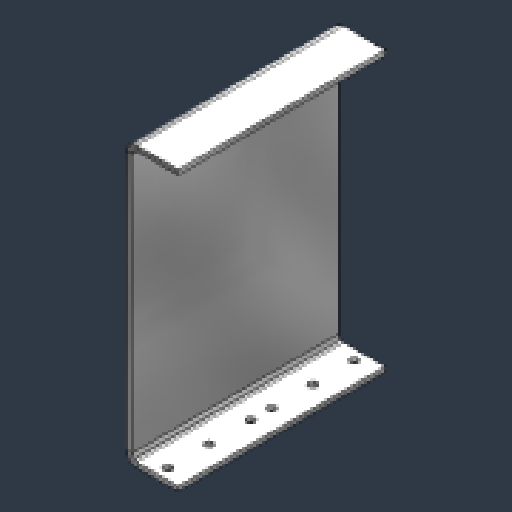
# Autodesk Inventor part: trough_back_support
Saved by Autodesk Inventor 2024.3 (Build 283343000, 343)
## iProperties
Created: 2025-03-03
Part Number: trough_back_support
Material: Aluminum 6061
Document SubType Name: Sheet Metal
Designer: marcu
Mass: 478.765 g
Surface Area: 1202.18 cm^2
Volume: 177.321 cm^3
Density: 2.7 g/cm^3
Sheet Metal Rule: Default
Appearance: Aluminum - Flat
Author: marcu
Autodesk Inventor part; units mm, degrees
ref_plane "YZ Plane" through (0, 0, 0) normal (1, 0, 0) x (0, 1, 0)
ref_plane "XZ Plane" through (0, 0, 0) normal (0, 1, 0) x (-1, 0, 0)
ref_plane "XY Plane" through (0, 0, 0) normal (0, 0, 1) x (1, 0, 0)
sketch "Sketch1" plane through (0, 0, 0) normal (0, 1, 0) x (-1, 0, 0)
  line L0 (-12.7, -63.5) -> (12.7, -63.5)
  line L1 (12.7, -63.5) -> (12.7, 63.5)
  line L2 (12.7, 63.5) -> (-12.7, 63.5)
  line L3 (-12.7, 63.5) -> (-12.7, -63.5)
  line L4 (-12.7, -63.5) -> (12.7, 63.5) construction
  line L5 (12.7, -63.5) -> (-12.7, 63.5) construction
  point P0 (0, 0)
  dimension "d0" = 25.4
  dimension "d1" = 127
  measures "d0" distance of L2.end L1.end
  measures "d1" distance of L0.end L1.end
extrude "Plate1" add sketch "Sketch1" along normal blind 3.048
sketch "Sketch2" plane through (-15.748, 6.096, 63.5) normal (-1, 0, 0) x (0, -1, 0)
  line L0 (0, -127) -> (0, 0)
  line L1 (0, 0) -> (-159.004, 0)
  line L2 (-159.004, 0) -> (-159.004, -127)
  line L3 (-159.004, -127) -> (0, -127)
  constraints: 6 end point, 1 horizontal, 1 perpendicular, 1 vertical
edge flange "Flange1" height 165.1 angle 90 thickness 3.048 bend radius 3.048 thickness toward (-1, 0, 0) relief straight relief width 3.048 relief depth 1.524 edges at (-12.7, 3.048, 0) wall of the first edge with corners at (-15.748, 6.096, -63.5) (-15.748, 6.096, 63.5) (-15.748, 165.1, 63.5) (-15.748, 165.1, -63.5)
bend "Bend1"
corner "Corner1"
sketch "Sketch3" plane through (0, 3.048, 0) normal (0, 1, 0) x (1, 0, 0)
  line L0 (-12.7, 63.5) -> (12.7, 63.5) construction
  line L1 (-12.7, -63.5) -> (-12.7, 63.5) construction
  line L2 (12.7, -63.5) -> (-12.7, -63.5) construction
  line L3 (12.7, 63.5) -> (12.7, -63.5) construction
  line L4 (12.7, 0) -> (-12.7, 0) construction
  point P0 (0, 0)
  point P1 (0, -6.35)
  point P2 (0, 0)
  point P3 (0, -31.75)
  point P4 (0, -57.15)
  point P5 (0, -82.55)
  point P6 (0, -107.95)
  point P7 (0, 6.35)
  point P8 (0, 31.75)
  point P9 (0, 57.15)
  point P10 (0, 82.55)
  point P11 (0, 107.95)
  dimension "d13" = 6.35
  dimension "d16" = 25.4
  dimension "d21" = 12.7
  constraints: 5 symmetric about line, 3 midpoint, 2 end point, 1 vertical, 4 other
  measures "d13" distance of point (0, 0) point (0, -6.35)
  measures "d16" distance of point (0, -6.35) point (0, -31.75)
  measures "d21" distance from line of L3 point (0, -6.35)
hole "Hole1" at (0, 3.048, 6.35) at (0, 3.048, 31.75) at (0, 3.048, 57.15) at (0, 3.048, 82.55) at (0, 3.048, -82.55) at (0, 3.048, -57.15) at (0, 3.048, -31.75) at (0, 3.048, -6.35) direction (0, -1, 0) diameter 5.1054 end through all clearance for "Flat Head Machine Screw (82)" size "#10" standard "Ansi Unified Screw Threads"
sketch "Sketch4" plane through (-12.7, 168.148, 63.5) normal (0, 1, 0) x (-1, 0, 0)
  line L0 (0, -127) -> (0, 0)
  line L1 (0, 0) -> (-25.4, 0)
  line L2 (-25.4, 0) -> (-25.4, -127)
  line L3 (-25.4, -127) -> (0, -127)
  constraints: 6 end point, 1 horizontal, 1 perpendicular, 1 vertical
edge flange "Flange2" height 31.496 angle 90 thickness 3.048 bend radius 3.048 thickness toward (0, 1, 0) relief straight relief width 3.048 relief depth 1.524 edges at (-15.748, 165.1, 0) wall of the first edge with corners at (-12.7, 168.148, -63.5) (-12.7, 168.148, 63.5) (12.7, 168.148, 63.5) (12.7, 168.148, -63.5)
bend "Bend2"
corner "Corner2"
sketch "Sketch5" plane through (12.7, 171.196, 63.5) normal (0, 1, 0) x (1, 0, 0)
  circle A0 centre (-12.7, 6.35) radius 2.5527 construction
  circle A1 centre (-12.7, 31.75) radius 2.5527 construction
  circle A2 centre (-12.7, 57.15) radius 2.5527 construction
  circle A3 centre (-12.7, 69.85) radius 2.5527 construction
  circle A4 centre (-12.7, 95.25) radius 2.5527 construction
  circle A5 centre (-12.7, 120.65) radius 2.5527 construction
  point P0 (-12.7, 63.5)
  constraints: 6 coincident
hole "Hole2" at (0, 171.196, 57.15) at (0, 171.196, 31.75) at (0, 171.196, 6.35) at (0, 171.196, -6.35) at (0, 171.196, -31.75) at (0, 171.196, -57.15) direction (0, -1, 0) diameter 5.1054 end through all clearance for "Flat Head Machine Screw (82)" size "#10" standard "Ansi Unified Screw Threads"
equation "\"d27\" = Thickness"
equation "\"d44\" = Thickness"
equation "\"d2\" = Thickness"
equation "\"d3\" = BendReliefWidth"
equation "\"d4\" = BendReliefDepth"
equation "\"d5\" = MinimumRemnant"
equation "\"d6\" = TransitionRadius"
equation "\"d9\" = BendRadius"
equation "\"d10\" = CornerReliefSize"
equation "\"d11\" = GapSize"
equation "\"d12\" = JacobiRadiusSize"
equation "\"d29\" = BendReliefWidth"
equation "\"d30\" = BendReliefDepth"
equation "\"d31\" = MinimumRemnant"
equation "\"d32\" = TransitionRadius"
equation "\"d35\" = BendRadius"
equation "\"d36\" = CornerReliefSize"
equation "\"d37\" = GapSize"
equation "\"d38\" = JacobiRadiusSize"
equation "\"BendRadius\" = Thickness"
equation "\"BendReliefWidth\" = Thickness"
equation "\"BendReliefDepth\" = 0.5 * Thickness"
equation "\"CornerReliefSize\" = 4 * Thickness"
equation "\"MinimumRemnant\" = 2 * Thickness"
equation "\"TransitionRadius\" = BendRadius"
equation "\"JacobiRadiusSize\" = BendRadius"
equation "\"GapSize\" = Thickness"
equation "\"Thickness\" = 3.048"
body "Solid1"
